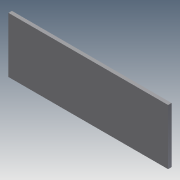
# Autodesk Inventor part: kinect rotate2 bottom
Saved by Autodesk Inventor 2011 (Build 150239000, 239)
## iProperties
Created: 2012-01-14
Part Number: kinect rotate2 bottom
Document SubType Name: Modeling
Designer: Matthew
Density: 1 g/cm^3
Author: Matthew
Autodesk Inventor part; units mm, degrees
ref_plane "YZ Plane" through (0, 0, 0) normal (1, 0, 0) x (0, 1, 0)
ref_plane "XZ Plane" through (0, 0, 0) normal (0, 1, 0) x (-1, 0, 0)
ref_plane "XY Plane" through (0, 0, 0) normal (0, 0, 1) x (1, 0, 0)
sketch "Sketch1" plane through (0, 0, 0) normal (0, 0, 1) x (1, 0, 0)
  line L0 (-39.9518, 9.6865) -> (252.1482, 9.6865)
  line L1 (252.1482, 9.6865) -> (252.1482, -91.9135)
  line L2 (252.1482, -91.9135) -> (-39.9518, -91.9135)
  line L3 (-39.9518, -91.9135) -> (-39.9518, 9.6865)
  point P0 (0, 0)
  dimension "d0" = 292.1
  dimension "d1" = 101.6
  constraints: 8 end point, 2 parallel, 1 horizontal, 1 perpendicular
  measures "d0" distance of L1.end L2.end
  measures "d1" distance of L0.end L1.end
extrude "Extrusion1" add sketch "Sketch1" along normal blind 6.35
body "Solid1"
